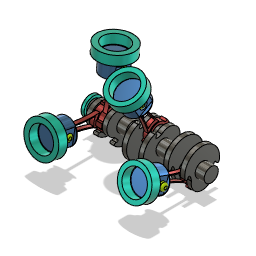
V6 Engine v2 (Autodesk Fusion 360 design; units mm, degrees)
Autodesk Fusion 360 part; units mm, degrees
note: some values were not read from the file. Set by a fixed rule: which sketch regions a step uses.
sketch "Sketch1" plane through (0, 0, 0) normal (1, 0, 0) x (0, 0, -1)
  line L0 (0, 0) -> (0, 50)
  line L1 (0, 50) -> (40, 50)
  line L2 (0, 0) -> (40, 0)
  line L3 (40, 50) -> (40, 48.5)
  line L4 (40, 48.5) -> (38, 48.5)
  line L5 (38, 48.5) -> (38, 47)
  line L6 (38, 47) -> (40, 47)
  line L7 (40, 47) -> (40, 45.5)
  line L8 (40, 45.5) -> (38, 45.5)
  line L9 (38, 45.5) -> (38, 44)
  line L10 (38, 44) -> (40, 44)
  line L11 (40, 44) -> (40, 42.5)
  line L12 (40, 42.5) -> (38, 42.5)
  line L13 (38, 42.5) -> (38, 41)
  line L14 (38, 41) -> (40, 41)
  line L15 (40, 50) -> (40, 48.5)
  line L16 (40, 41) -> (40, 0)
  dimension "d1" = 50
  dimension "d2" = 40
  dimension "d3" = 50
  dimension "d4" = 1.5
  dimension "d5" = 2
  dimension "d6" = 1.5
  dimension "d7" = 1.5
  dimension "d8" = 1.5
  constraint coincident L0.start L2.start
  constraint vertical L0
  constraint perpendicular L0 L1
  constraint perpendicular L1 L15
  constraint perpendicular L1 L3
  constraint perpendicular L3 L4
  constraint perpendicular L4 L5
  constraint coincident L6.end L15
  constraint perpendicular L6 L15
  constraint perpendicular L6 L7
  constraint perpendicular L7 L8
  constraint perpendicular L8 L9
  constraint coincident L10.end L15
  constraint perpendicular L10 L15
  constraint perpendicular L10 L11
  constraint perpendicular L12 L15
  constraint perpendicular L12 L13
  constraint coincident L14.end L15
  constraint perpendicular L14 L15
  measures "d1" distance of L0.start L0.end
  measures "d2" distance of L0.end L1.end
  measures "d3" distance of L1.end L2.end
  measures "d4" distance of L1.end L3.end
  measures "d5" distance of L3.end L4.end
  measures "d6" distance of L4.end L5.end
  measures "d7" distance of L6.end L7.end
  measures "d8" distance of L10.end L11.end
revolve "Revolve1" add sketch "Sketch1" angle 360 about axis through (0, 0, 0) along (0, 1, 0) makes body 1 in component "Piston1"
sketch "Sketch2" plane through (0, 0, 0) normal (1, 0, 0) x (0, 0, -1)
  line L0 (0, -10) -> (0, 60)
  circle A0 centre (0, 18.596) radius 12.5
  line L1 (-40, 0) -> (40, 0)
  dimension "d10" = 25
  dimension "d11" = 18.596
  constraint vertical L0
  constraint coincident L0 A0.centre
  measures "d10" diameter of A0
  measures "d11" distance of A0.centre L1
extrude "Extrude1" cut sketch "Sketch2" along normal mid plane 90 bodies 1 in component "Piston1"
sketch "Sketch3" plane through (0, 0, 0) normal (0, 0, 1) x (1, 0, 0)
  line L0 (40, 0) -> (30.861, 0)
  line L1 (30.861, 0) -> (30.861, 36)
  line L2 (45, 2.6326) -> (45, 2)
  line L3 (0, 0) -> (0, 52.3643)
  line L4 (-30.861, 0) -> (-30.861, 36)
  line L5 (-30.861, 36) -> (-45, 36)
  line L6 (-45, 36) -> (-45, 2)
  line L7 (-45, 2.6326) -> (-30.861, 2.6326)
  line L8 (30.861, 36) -> (42, 36)
  line L9 (42, 36) -> (42, 2)
  line L10 (42, 2) -> (30.861, 2)
  dimension "d14" = 9.139
  constraint horizontal L0
  constraint perpendicular L0 L1
  constraint perpendicular L0 L2
  constraint coincident L3.start origin
  constraint vertical L3
  constraint symmetric L0.end L3 L4.start
  constraint symmetric L1.end L3 L4.end
  constraint symmetric L2.end L3 L6.end
  constraint symmetric L2.start L3 L7.start
  constraint perpendicular L1 L8
  constraint perpendicular L8 L9
  constraint coincident L1 L10.end
  constraint perpendicular L1 L10
  measures "d14" distance of L0.start L0.end
extrude "Extrude2" cut sketch "Sketch3" along normal mid plane 220 bodies 1 in component "Piston1"
sketch "Sketch4" plane through (0, 0, 0) normal (0, -1, 0) x (1, 0, 0)
  circle A0 centre (0, 0) radius 40
  circle A1 centre (0, 0) radius 30
  line L0 (20.661, 32.8772) -> (20.661, -33.0603)
  line L1 (0, 30) -> (0, 0) construction
  line L2 (-20.661, 32.8772) -> (-20.661, -33.0603)
  dimension "d17" = 60
  dimension "d18" = 20.661
  constraint coincident A0.centre A1.centre
  constraint vertical L0
  constraint coincident A1 L1.start
  constraint parallel L0 L1
  constraint symmetric L0.start L1 L2.start
  constraint symmetric L0.end L1 L2.end
  measures "d17" diameter of A1
  measures "d18" distance of L0 L1
extrude "Extrude3" cut sketch "Sketch4" against normal blind 37 contours A1 L0 L2 bodies 1 in component "Piston1"
sketch "Sketch5" plane through (0, 0, 0) normal (1, 0, 0) x (0, 0, -1)
  circle A0 centre (0, 0) radius 12.5
  circle A1 centre (0, 0) radius 16.0015
  line L0 (0, 0) -> (0, -151.095)
  circle A2 centre (0, -151.095) radius 23.4205
  circle A3 centre (0, -151.095) radius 31.5
  spline S0 degree 5 poles (11.9641, -10.6259) (11.6197, -18.2759) (11.1233, -32.6974) (10.9554, -51.6965) (11.7258, -72.4887) (13.7917, -93.4423) (15.9857, -107.7333) (17.8356, -117.5179) (19.1539, -123.653) (19.8343, -126.6235) knots 0 0 0 0 0 0 0.2 0.4 0.6 0.8 1 1 1 1 1 1
  line L1 (12.8511, 9.0794) -> (11.077, -30.3312)
  spline S1 degree 5 poles (-11.9641, -10.6259) (-11.6197, -18.2759) (-11.1233, -32.6974) (-10.9554, -51.6965) (-11.7258, -72.4887) (-13.7917, -93.4423) (-15.9857, -107.7333) (-17.8356, -117.5179) (-19.1539, -123.653) (-19.8343, -126.6235) knots 0 0 0 0 0 0 0.2 0.4 0.6 0.8 1 1 1 1 1 1
  line L2 (18.0869, -118.9948) -> (21.5816, -134.2523)
  line L3 (-12.8511, 9.0794) -> (-11.077, -30.3312)
  line L4 (-18.0869, -118.9948) -> (-21.5816, -134.2523)
  spline S2 degree 3 poles (-8.9671, -10.491) (-8.924, -11.4476) (-8.8828, -12.3958) (-8.8434, -13.3357) knots 0 0 0 0 0.014958 0.014958 0.014958 0.014958
  spline S3 degree 3 poles (8.9671, -10.491) (8.924, -11.4476) (8.8828, -12.3958) (8.8434, -13.3357) knots 0 0 0 0 0.014958 0.014958 0.014958 0.014958
  arc A4 (-8.6593, -18.0282) -> (8.6593, -18.0282) centre (0, 0) ccw
  arc A5 (17.0971, -113.2804) -> (-13.8107, -111.9604) centre (0, -151.095) ccw
  spline S4 degree 3 poles (-8.6593, -18.0282) (-8.2455, -29.368) (-8.1074, -39.4585) (-8.2021, -48.4973) (-8.3646, -64.0091) (-9.1923, -76.518) (-10.3558, -87.5004) (-11.3133, -96.5383) (-12.4951, -104.5522) (-13.8107, -111.9604) knots 0.040223 0.040223 0.040223 0.040223 0.226146 0.226146 0.226146 0.545211 0.545211 0.545211 0.807787 0.807787 0.807787 0.807787
  spline S5 degree 3 poles (8.6593, -18.0282) (8.2455, -29.368) (8.1074, -39.4585) (8.2021, -48.4973) (8.3646, -64.0091) (9.1923, -76.518) (10.3558, -87.5004) (11.3133, -96.5383) (12.4951, -104.5522) (13.8107, -111.9604) knots 0.040223 0.040223 0.040223 0.040223 0.226146 0.226146 0.226146 0.545211 0.545211 0.545211 0.807787 0.807787 0.807787 0.807787
  dimension "d21" = 25
  dimension "d22" = 32.003
  dimension "d23" = 151.095
  dimension "d24" = 46.841
  dimension "d29" = 63
  dimension "d32" = 40
  dimension "d33" = 83
  constraint coincident A0.centre A1.centre
  constraint vertical L0
  constraint coincident L0.end A2.centre
  constraint concentric A2 A3
  constraint coincident A1 S0.start
  constraint coincident A3 S0.end
  constraint midpoint S0.start L1
  constraint midpoint S0.end L2
  constraint symmetric L0 S0.start S1.start
  constraint symmetric L0 S0.end S1.end
  constraint symmetric L0 L1.start L3.start
  constraint symmetric L0 L1.end L3.end
  constraint symmetric L0 L2.start L4.start
  constraint symmetric L0 L2.end L4.end
  constraint concentric A3 A5
  constraint coincident A1 S2.end
  constraint coincident A1 S3.end
  constraint coincident S0 A5.start
  constraint coincident A5 S5.end
  measures "d21" diameter of A0
  measures "d22" diameter of A1
  measures "d23" distance of A0.centre L0.end
  measures "d24" diameter of A2
  measures "d29" diameter of A3
  measures "d32" diameter of A4
  measures "d33" diameter of A5
extrude "Extrude1'" add sketch "Sketch5" along normal mid plane 20 separate body contours A0 A1 L1 L3 | A0 A1 L0 L1 | A0 A1 L0 L3 | A3 makes body 2 at (6.6667, -0.7976, -15.9816) makes body 3 at (3.3333, -147.9586, -31.3435) in component "Connecting rod 1"
extrude "Extrude2'" add sketch "Sketch5" along normal mid plane 14 contours A1 L0 S0 A4 A5 S5 | A1 L0 A3 S1 A4 A5 S4 | L0 A3 S0 A5 bodies 2 3 in component "Connecting rod 1"
sketch "Sketch7" plane through (0, 0, 0) normal (1, 0, 0) x (0, 0, -1)
  line L0 (30.5621, -143.4673) -> (38, -143.4673)
  line L1 (38, -143.4673) -> (38, -151)
  line L2 (30.5621, -158.5327) -> (38, -158.5327)
  line L3 (38, -158.5327) -> (38, -151)
  line L4 (-30.5621, -143.4673) -> (-38, -143.4673)
  line L5 (-38, -143.4673) -> (-38, -151)
  line L6 (-38, -158.5327) -> (-38, -151)
  line L7 (-30.5621, -158.5327) -> (-38, -158.5327)
  arc A0 (-30.5621, -143.4673) -> (-30.5621, -158.5327) centre (0, -151) ccw
  arc A1 (30.5621, -158.5327) -> (30.5621, -143.4673) centre (0, -151) ccw
  constraint horizontal L0
  constraint coincident L2.start A0
  constraint concentric A0 A1
extrude "Extrude3'" add sketch "Sketch7" along normal mid plane 20 bodies 2 in component "Connecting rod 1"
sketch "Sketch8" plane through (0, 0, 0) normal (1, 0, 0) x (0, 0, -1)
  circle A0 centre (0, 0) radius 23.4205
  circle A1 centre (0, 0) radius 36.1865
  line L0 (0, 0) -> (0, -32.692)
  spline S0 degree 5 poles (35.4531, -7.2484) (35.6528, -8.3553) (36.0539, -10.4799) (36.6615, -13.3987) (37.4866, -16.7664) (38.5608, -20.1542) (39.6976, -22.7662) (40.9104, -24.6259) (42.1964, -25.7261) (43.5281, -26.0283) (44.8346, -25.4717) (45.7841, -24.2801) (46.4051, -22.935) (46.7732, -21.8325) (46.9458, -21.2299) knots 0 0 0 0 0 0 0.1 0.2 0.3 0.4 0.5 0.6 0.7 0.8 0.9 1 1 1 1 1 1
  spline S1 degree 5 poles (-35.4531, -7.2484) (-35.6561, -8.3737) (-36.0642, -10.5338) (-36.6832, -13.5024) (-37.5254, -16.9281) (-38.6228, -20.3641) (-39.7833, -22.9874) (-41.0191, -24.8094) (-42.327, -25.8149) (-43.6796, -25.9659) (-45.0088, -25.2169) (-45.984, -23.8565) (-46.6315, -22.3854) (-47.0211, -21.2006) (-47.2054, -20.5571) knots 0 0 0 0 0 0 0.1 0.2 0.3 0.4 0.5 0.6 0.7 0.8 0.9 1 1 1 1 1 1
  line L1 (34.5242, -2.0972) -> (36.3821, -12.3995)
  line L2 (45.7439, -25.4246) -> (48.6123, -15.4072)
  line L3 (-34.5242, -2.0972) -> (-36.3821, -12.3995)
  line L4 (-45.7439, -25.4246) -> (-48.6123, -15.4072)
  arc A2 (-56.6372, -21.7395) -> (56.6372, -21.7395) centre (0, -32.692) ccw
  arc A3 (-47.2054, -20.5571) -> (-56.6372, -21.7395) centre (-51.7282, -22.6888) ccw
  arc A4 (56.6372, -21.7395) -> (46.9458, -21.2299) centre (51.7282, -22.6888) ccw
  point P0 (42.5686, -25.688)
  point P1 (-42.5686, -25.688)
  dimension "d40" = 46.841
  dimension "d41" = 72.373
  dimension "d42" = 32.692
  dimension "d43" = 115.373
  dimension "d44" = 5
  constraint coincident A0.centre A1.centre
  constraint concentric A0 A1
  constraint vertical L0
  constraint coincident L0.end A2.centre
  constraint coincident A1 S0.start
  constraint midpoint S0.start L1
  constraint symmetric L0 S0.start S1.start
  constraint symmetric L0 P0 P1
  constraint symmetric L0 L1.start L3.start
  constraint symmetric L0 L1.end L3.end
  constraint symmetric L0 L2.start L4.start
  constraint symmetric L0 L2.end L4.end
  constraint tangent A2 A3
  constraint tangent S1 A3
  constraint tangent S0 A4
  constraint tangent A2 A4
  constraint equal A3 A4
  measures "d40" diameter of A0
  measures "d41" diameter of A1
  measures "d42" distance of A0.centre L0.end
  measures "d43" diameter of A2
  measures "d44" radius of A3
extrude "Extrude1''" add sketch "Sketch8" against normal blind 15 separate body contours A0 | A1 | A1 S0 S1 A2 A3 A4 makes body 4
extrude "Extrude2''" add sketch "Sketch8" along normal blind 40 contours A0 bodies 4
extrude "Extrude3''" add sketch "Sketch8" along normal blind 15 from surface at 40 contours A0 | A1 | A1 S0 S1 A2 A3 A4 bodies 4
sketch "Sketch9" plane through (55, 0, 0) normal (1, 0, 0) x (0, 0, -1)
  arc A0 (35.4531, -7.2484) -> (-35.4531, -7.2484) centre (0, 0) ccw
  spline S0 degree 5 poles (-35.4531, -7.2484) (-35.6561, -8.3737) (-36.0642, -10.5338) (-36.6832, -13.5024) (-37.5254, -16.9281) (-38.6228, -20.3641) (-39.7833, -22.9874) (-41.0191, -24.8094) (-42.327, -25.8149) (-43.6796, -25.9659) (-45.0088, -25.2169) (-45.984, -23.8565) (-46.6315, -22.3854) (-47.0211, -21.2006) (-47.2054, -20.5571) knots 0 0 0 0 0 0 0.1 0.2 0.3 0.4 0.5 0.6 0.7 0.8 0.9 1 1 1 1 1 1
  arc A1 (-47.2054, -20.5571) -> (-56.6372, -21.7395) centre (-51.7282, -22.6888) ccw
  arc A2 (-56.6372, -21.7395) -> (56.6372, -21.7395) centre (0, -32.692) ccw
  arc A3 (56.6372, -21.7395) -> (46.9458, -21.2299) centre (51.7282, -22.6888) ccw
  spline S1 degree 5 poles (46.9458, -21.2299) (46.7732, -21.8325) (46.4051, -22.935) (45.7841, -24.2801) (44.8346, -25.4717) (43.5281, -26.0283) (42.1964, -25.7261) (40.9104, -24.6259) (39.6976, -22.7662) (38.5608, -20.1542) (37.4866, -16.7664) (36.6615, -13.3987) (36.0539, -10.4799) (35.6528, -8.3553) (35.4531, -7.2484) knots -1 -1 -1 -1 -1 -1 -0.9 -0.8 -0.7 -0.6 -0.5 -0.4 -0.3 -0.2 -0.1 0 0 0 0 0 0
  circle A4 centre (-0.0479, -23.2801) radius 23.4205
  dimension "d52" = 46.841
  measures "d52" diameter of A4
extrude "Extrude4" add sketch "Sketch9" along normal blind 30 contours A4 bodies 4
ref_plane "WorkPlane1" through (20, -29.208, 0) normal (1, 0, 0) x (0, 0, -1)
mirror "Mirror1" about plane through (20, -29.208, 0) normal (1, 0, 0) of "Extrude4"
move_body "Move1" bodies 4 to x (1, 0, 0) y (0, 1, 0) z (0, 0, 1) at (-55.603, 0, 4.3163)
copy_body "Body->Comp1" bodies 4 removing the originals makes body 5 in component "Crank"
copy_body "CopyPasteBodies1" bodies 5 makes body 6 in component "Crank"
move_body "Move1'" bodies 6 to x (1, 0, 0) y (0, -0.5, -0.866025) z (0, 0.866025, -0.5) at (130, -38.6997, -13.6148) in component "Crank"
copy_body "CopyPasteBodies2" bodies 6 makes body 7 in component "Crank"
move_body "Move2" bodies 7 to x (1, 0, 0) y (0, -0.5, -0.866025) z (0, 0.866025, -0.5) at (-260, -38.6997, -13.6148) in component "Crank"
sketch "Sketch10" plane through (-427.8511, 0, 0) normal (-1, 0, 0) x (0, 0, 1)
  line L0 (84.7716, 45.3368) -> (84.7716, 78.7043)
  line L1 (84.7716, 78.7043) -> (33.8757, 78.7043)
  line L2 (33.8757, 78.7043) -> (33.8757, 45.3368)
  line L3 (33.8757, 45.3368) -> (84.7716, 45.3368)
  circle A0 centre (59.3236, 61.3003) radius 12.5
  circle A1 centre (59.3236, 61.3003) radius 12.5
  constraint concentric A0 A1
extrude "Extrude1'''" add sketch "Sketch10" against normal up to surface (61.722 mm away) separate body contours A0 A1 makes body 8 in component "Piston pin"
extrude "Extrude2'''" add 1 faces at (-427.8511, 56.8873, 60.7654) along direction (-1, 0, 0) blind 5 on bodies 8 bodies 8 in component "Piston pin"
extrude "Extrude3'''" add 1 faces at (-366.1291, 64.1012, 59.7558) along direction (1, 0, 0) blind 5 on bodies 8 bodies 8 in component "Piston pin"
fillet "Fillet1" radius 7.5 2 edges at (-361.1291, 65.8205, 47.6696) (-432.8511, 56.7801, 47.6696) 1 faces at (-361.1291, 56.8873, 60.7654) on bodies 8 in component "Piston pin"
sketch "Sketch11" plane through (-223.9524, 0, 0) normal (-1, 0, 0) x (0, 0, 1)
  circle A0 centre (2.455, -5.7325) radius 23.4205
  circle A1 centre (2.455, -5.7325) radius 31.7146
  constraint concentric A0 A1
extrude "Extrude1''''" add sketch "Sketch11" along normal blind 10 separate body makes body 9 in component "Component"
sketch "Sketch12" plane through (0, 39.5163, 224.1079) normal (0, 0.173648, 0.984808) x (1, 0, 0)
  circle A0 centre (-229.2333, -11.8559) radius 40
  circle A1 centre (-229.2333, -11.8559) radius 57.0732
  constraint concentric A0 A1
extrude "Extrude1'''''" add sketch "Sketch12" along normal blind 30 separate body makes body 10 in component "Component'"
sketch "Sketch13" plane through (0, 173.9515, -15.2188) normal (0, 0.996195, -0.087156) x (-1, 0, 0)
  circle A0 centre (210.5553, 45.9279) radius 40
  circle A1 centre (210.5553, 45.9279) radius 58.1108
  constraint concentric A0 A1
extrude "Extrude1''''''" add sketch "Sketch13" along normal blind 30 separate body makes body 11 in component "Component''"
sketch "Sketch14" plane through (0, 66.3472, 182.2875) normal (0, 0.34202, 0.939693) x (1, 0, 0)
  circle A0 centre (50.7667, -45.4836) radius 40
  circle A1 centre (50.7667, -45.4836) radius 54.3687
  constraint concentric A0 A1
extrude "Extrude1'''''''" add sketch "Sketch14" along normal blind 30 separate body makes body 12 in component "Component'''"
sketch "Sketch15" plane through (0, 157.7481, 91.0759) normal (0, 0.866025, 0.5) x (1, 0, 0)
  circle A0 centre (-95.5553, -7.2647) radius 40
  circle A1 centre (-95.5553, -7.2647) radius 54.4699
  constraint concentric A0 A1
extrude "Extrude1''''''''" add sketch "Sketch15" along normal blind 30 separate body makes body 13 in component "Component''''"
component "Piston1" placed x (1, 0, 0) y (0, 0.34202, 0.939693) z (0, -0.939693, 0.34202) at (50.7667, 6.5056, 150.8591)
component "Connecting rod 1" placed x (1, 0, 0) y (0, 0.34202, 0.939693) z (0, -0.939693, 0.34202) at (50.1057, 12.8658, 168.3337)
component "Crank" placed x (1, 0, 0) y (0, 0.5, -0.866025) z (0, 0.866025, 0.5) at (-54.2913, -7.6711, 3.9597)
component "Piston pin" placed x (1, 0, 0) y (0, 0.984808, -0.173648) z (0, 0.173648, 0.984808) at (167.0958, -48.2832, 147.462)
component "Piston1" placed x (1, 0, 0) y (0, 0.173648, 0.984808) z (0, -0.984808, 0.173648) at (-229.2333, 19.1581, 176.9262)
component "Piston1" placed x (1, 0, 0) y (0, 0.996195, -0.087156) z (0, 0.087156, 0.996195) at (-210.5553, 128.1447, 34.8921)
component "Piston1" placed x (1, 0, 0) y (0, 0.866025, 0.5) z (0, -0.5, 0.866025) at (-95.5553, 110.8145, 72.3674)
component "Connecting rod 1" placed x (1, 0, 0) y (0, 0.996195, -0.087156) z (0, 0.087156, 0.996195) at (-209.8943, 146.6699, 33.2714)
component "Connecting rod 1" placed x (1, 0, 0) y (0, 0.173648, 0.984808) z (0, -0.984808, 0.173648) at (-229.8943, 22.3872, 195.2397)
component "Connecting rod 1" placed x (1, 0, 0) y (0, 0.866025, 0.5) z (0, -0.5, 0.866025) at (-99.8943, 126.9191, 81.6654)
component "Component" placed x (1, 0, 0) y (0, 1, 0) z (0, 0, 1) at (-60.9419, -9.7991, 23.848)
component "Component'" placed x (1, 0, 0) y (0, 1, 0) z (0, 0, 1) at (0, 0, 0)
component "Component''" placed x (1, 0, 0) y (0, 1, 0) z (0, 0, 1) at (0, 0, 0)
component "Component'''" placed x (1, 0, 0) y (0, 1, 0) z (0, 0, 1) at (0, 0, 0)
component "Component''''" placed x (1, 0, 0) y (0, 1, 0) z (0, 0, 1) at (0, 0, 0)
component "Piston pin" placed x (1, 0, 0) y (0, 0.939693, -0.34202) z (0, 0.34202, 0.939693) at (457.0958, -65.0275, 133.5536)
component "Piston pin" placed x (1, 0, 0) y (0, 0.866025, 0.5) z (0, -0.5, 0.866025) at (297.0958, 103.4933, -0.3606)
component "Piston pin" placed x (1, 0, 0) y (0, 0.996195, -0.087156) z (0, 0.087156, 0.996195) at (185.7738, 80.4325, -20.4838)
equation "d10 = ( 12.5 * 2 ) * 1 mm"
